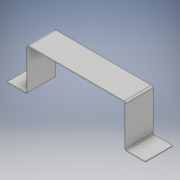
# Autodesk Inventor part: batteryHolder
Saved by Autodesk Inventor 2017 (Build 210142000, 142)
## iProperties
Created: 2017-02-09
Part Number: batteryHolder
Material: Generic
Document SubType Name: Sheet Metal
Designer: kingb
Density: 1 g/cm^3
Sheet Metal Rule: Default
Appearance: Default
Author: kingb
Autodesk Inventor part; units mm, degrees
ref_plane "YZ Plane" through (0, 0, 0) normal (1, 0, 0) x (0, 1, 0)
ref_plane "XZ Plane" through (0, 0, 0) normal (0, 1, 0) x (-1, 0, 0)
ref_plane "XY Plane" through (0, 0, 0) normal (0, 0, 1) x (1, 0, 0)
sketch "Sketch1" plane through (0, 0, 0) normal (0, 1, 0) x (-1, 0, 0)
  line L0 (0, 0) -> (180.975, 0)
  line L1 (180.975, 0) -> (180.975, -50.8)
  line L2 (180.975, -50.8) -> (0, -50.8)
  line L3 (0, -50.8) -> (0, 0)
  dimension "d0" = 180.975
  dimension "d1" = 50.8
  measures "d0" distance of L1.end L2.end
  measures "d1" distance of L0.end L1.end
extrude "Plate1" add sketch "Sketch1" along normal blind 1.5875
sketch "Sketch2" plane through (0, 0, 0) normal (1, 0, 0) x (0, 1, 0)
  line L0 (0, -50.8) -> (0, 0)
  line L1 (0, 0) -> (-76.0603, 0)
  line L2 (-76.0603, 0) -> (-76.0603, -50.8)
  line L3 (-76.0603, -50.8) -> (0, -50.8)
  constraints: 6 end point, 1 horizontal, 1 perpendicular, 1 vertical
edge flange "Flange1" height 77.6478 angle 90 thickness 1.5875 bend radius 1.5875 thickness toward (1, 0, 0) relief straight relief width 1.5875 relief depth 0.7937 corner gap 1.5875 corner form 0 edges at (0, 0, -25.4) (-180.975, 0, -25.4) wall of the first edge with corners at (0, 0, -50.8) (0, 0, 0) (0, -76.0603, 0) (0, -76.0603, -50.8)
bend "Bend1"
corner "Corner1"
sketch "Sketch3" plane through (1.5875, -76.0603, -50.8) normal (0, -1, 0) x (1, 0, 0)
  line L0 (0, 50.8) -> (0, 0)
  line L1 (0, 0) -> (36.5125, 0)
  line L2 (36.5125, 0) -> (36.5125, 50.8)
  line L3 (36.5125, 50.8) -> (0, 50.8)
  constraints: 6 end point, 1 horizontal, 1 perpendicular, 1 vertical
edge flange "Flange2" height 38.1 angle 90 thickness 1.5875 bend radius 1.5875 thickness toward (0, -1, 0) relief straight relief width 1.5875 relief depth 0.7937 corner gap 1.5875 corner form 0 edges at (1.5875, -76.0603, -25.4) (-182.5625, -76.0603, -25.4) wall of the first edge with corners at (1.5875, -76.0603, 0) (1.5875, -76.0603, -50.8) (38.1, -76.0603, -50.8) (38.1, -76.0603, 0)
bend "Bend2"
corner "Corner2"
equation "\"d3\" = BendReliefWidth"
equation "\"d4\" = BendReliefDepth"
equation "\"d5\" = MinimumRemnant"
equation "\"d6\" = BendRadius"
equation "\"d9\" = BendRadius"
equation "\"d10\" = CornerReliefSize"
equation "\"d11\" = GapSize"
equation "\"d12\" = JacobiRadiusSize"
equation "\"d13\" = BendReliefWidth"
equation "\"d14\" = BendReliefDepth"
equation "\"d15\" = MinimumRemnant"
equation "\"d16\" = BendRadius"
equation "\"d19\" = BendRadius"
equation "\"d20\" = CornerReliefSize"
equation "\"d21\" = GapSize"
equation "\"d22\" = JacobiRadiusSize"
equation "\"BendRadius\" = Thickness"
equation "\"BendReliefWidth\" = Thickness"
equation "\"BendReliefDepth\" = 0.5 * Thickness"
equation "\"CornerReliefSize\" = 4 * Thickness"
equation "\"MinimumRemnant\" = 2 * Thickness"
equation "\"TransitionRadius\" = BendRadius"
equation "\"JacobiRadiusSize\" = Thickness"
equation "\"GapSize\" = Thickness"
equation "\"d2\" = BendRadius"
equation "\"Thickness\" = 1.5875"
body "Solid1"
